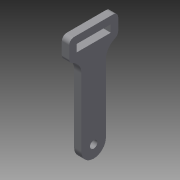
# Autodesk Inventor part: 27030914CameraMountA-2
Saved by Autodesk Inventor 2015 (Build 190159000, 159)
## iProperties
Created: 2013-05-28
Part Number: 27030914CameraMountA-2
Material: Generic
Document SubType Name: Modeling
Designer: Eric
Density: 1 g/cm^3
Appearance: Default
Author: Eric
Autodesk Inventor part; units mm, degrees
ref_plane "YZ Plane" through (0, 0, 0) normal (1, 0, 0) x (0, 1, 0)
ref_plane "XZ Plane" through (0, 0, 0) normal (0, 1, 0) x (-1, 0, 0)
ref_plane "XY Plane" through (0, 0, 0) normal (0, 0, 1) x (1, 0, 0)
sketch "Sketch1" plane through (0, 0, 0) normal (1, 0, 0) x (0, 1, 0)
  line L0 (-8.7654, 33.1522) -> (-8.7039, 33.1268)
  line L1 (8.7039, 33.1268) -> (8.7654, 33.1522)
  line L2 (-5, 27.5835) -> (-5, 0)
  line L3 (5, 27.5835) -> (5, 0)
  arc A0 (-5, 27.5835) -> (-8.7039, 33.1268) centre (-11, 27.5835) ccw
  arc A1 (8.7039, 33.1268) -> (5, 27.5835) centre (11, 27.5835) ccw
  line L4 (-7, 36) -> (7, 36)
  line L5 (-10, 36) -> (-10, 35)
  line L6 (10, 36) -> (10, 35)
  circle A2 centre (0, 0) radius 46 construction
  arc A3 (-10, 35) -> (-8.7654, 33.1522) centre (-8, 35) ccw
  arc A4 (8.7654, 33.1522) -> (10, 35) centre (8, 35) ccw
  circle A5 centre (0, 0) radius 1.5
  arc A6 (-5, 0) -> (5, 0) centre (0, 0) ccw
  line L7 (0, 0) -> (0, 36) construction
  line L8 (-10, 36) -> (-9.7321, 36)
  line L9 (10, 42) -> (-10, 42)
  line L10 (-10, 42) -> (-10, 36)
  line L11 (10, 36) -> (9.7321, 36)
  line L12 (10, 42) -> (10, 36)
  line L13 (-7, 36) -> (-7, 39)
  line L14 (-7, 39) -> (7, 39)
  line L15 (7, 39) -> (7, 36)
  point P0 (-5, 31.5926)
  point P1 (5, 31.5926)
  dimension "d25" = 10
  dimension "d32" = 6
  dimension "d33" = 6
  dimension "d82" = 46
  dimension "d90" = 2
  dimension "d93" = 1
  dimension "d95" = 22.5
  dimension "d109" = 3
  dimension "d112" = 36
  dimension "d113" = 5
  dimension "d115" = 20
  dimension "d118" = 6
  dimension "d120" = 6
  constraints: 32 end point, 12 point on circle, 8 tangent, 7 centre point, 7 coincident, 4 point on line, 3 horizontal, 3 parallel, 3 vertical, 2 perpendicular, 2 vertical alignment, 1 concentric, 1 equal radius, 1 midpoint, 2 other
  measures "d25" distance between parallel lines of L2 L3
  measures "d32" radius of A0
  measures "d33" radius of A1
  measures "d82" radius of A2
  measures "d90" radius of A3
  measures "d93" distance from line of L4 A3.centre
  measures "d95" angle of L0 L4
  measures "d109" diameter of A5
  measures "d112" distance from line of point (0, 0) L4
  measures "d113" radius of A6
  measures "d115" distance of L5.start L6.start
  measures "d118" distance of L9.end L5.start
  measures "d120" distance of L9.start L6.start
extrude "Extrusion10" add sketch "Sketch1" along normal blind 3
fillet "Fillet1" radius 2 2 edges at (1.5, -10, 42) (1.5, 10, 42)
body "Solid10"
